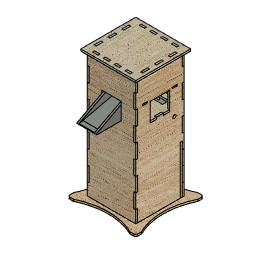
Plant fountain v41 (Autodesk Fusion 360 design; units mm, degrees)
Autodesk Fusion 360 part; units mm, degrees
(part 1 of 3)
sketch "base" plane through (0, 0, 0) normal (0, 0, 1) x (1, 0, 0) in component "base"
  line L0 (0, 0) -> (75, 0)
  line L1 (75, 0) -> (75, 75)
  line L2 (75, 75) -> (0, 75)
  line L3 (0, 75) -> (0, 0)
  line L4 (75, 37.5) -> (0, 37.5) construction
  line L5 (37.5, 75) -> (37.5, 0) construction
  line L6 (-5, 80) -> (80, 80)
  line L7 (80, 80) -> (80, -5)
  line L8 (80, -5) -> (-5, -5)
  line L9 (-5, -5) -> (-5, 80)
  line L10 (-5, 80) -> (80, -5) construction
  line L11 (80, 80) -> (-5, -5) construction
  point P0 (37.5, 37.5)
  dimension "d14" = 75
  dimension "d15" = 75
  dimension "d16" = 5
  dimension "d17" = 5
  constraint horizontal L0
  constraint vertical L1
  constraint horizontal L2
  constraint vertical L3
  constraint coincident L0.start L3.end
  constraint midpoint L1 L4.start
  constraint midpoint L3 L4.end
  constraint midpoint L2 L5.start
  constraint midpoint L0 L5.end
  constraint horizontal L6
  constraint perpendicular L6 L7
  constraint parallel L6 L8
  constraint parallel L7 L9
  constraint coincident L10 P0
  constraint coincident L11 P0
  constraint midpoint L4 P0
  measures "d14" distance of L1.end L2.end
  measures "d15" distance of L0.end L1.end
  measures "d16" distance of L2 L6
  measures "d17" distance of L1 L7
extrude "Extrude1" add sketch "base" along normal blind 3 contours L0 L1 L2 L3 | L6 L7 L8 L9 makes body 1 in component "base"
sketch "lenghttabcut" plane through (0, 0, 3) normal (0, 0, 1) x (-1, 0, 0) in component "base"
  line L0 (5, 5) -> (-80, 5)
  line L1 (-80, 5) -> (-80, -80)
  line L2 (-80, -80) -> (5, -80)
  line L3 (5, -80) -> (5, 5)
  line L4 (-8.3333, -75) -> (-16.6667, -75)
  line L5 (-16.6667, -75) -> (-16.6667, -72)
  line L6 (-16.6667, -72) -> (-8.3333, -72)
  line L7 (-8.3333, -72) -> (-8.3333, -75)
  line L8 (-75, -75) -> (0, -75)
  line L9 (0, -75) -> (0, 0)
  dimension "d20" = 8.3333
  dimension "d21" = 8.3333
  dimension "d35" = 3
  constraint horizontal L4
  constraint vertical L5
  constraint horizontal L6
  constraint vertical L7
  constraint collinear L4 L8
  measures "d20" distance of L7 L9
  measures "d21" distance of L4.start L4.end
  measures "d35" distance of L4.start L6.end
extrude "Extrude2" cut sketch "lenghttabcut" against normal blind 3 contours L4 L5 L6 L7 L8 bodies 1 in component "base"
pattern_linear "R-Pattern1" count 4 spacing 16.6667 along (1, 0, 0) of "Extrude2" in component "base"
ref_plane "WorkPlane1" through (37.5, 75, 1.5) normal (0, 1, 0) x (-1, 0, 0) in component "back"
sketch "back" plane through (30, 75, 1.5) normal (0, 1, 0) x (1, 0, 0) in component "back"
  line L0 (-30, 1.5) -> (45, 1.5)
  line L1 (45, 1.5) -> (45, -198.5)
  line L2 (45, -198.5) -> (-30, -198.5)
  line L3 (-30, -198.5) -> (-30, 1.5)
  point P0 (7.5, 1.5)
  dimension "d29" = 200
  dimension "d30" = 75
  constraint horizontal L0
  constraint vertical L1
  constraint horizontal L2
  constraint vertical L3
  constraint midpoint L0 P0
  measures "d29" distance of L0.start L2.end
  measures "d30" distance of L1.end L2.end
extrude "Extrude1'" add sketch "back" against normal blind 3 separate body makes body 2 in component "back"
sketch "heighttabcut" plane through (75, 0, 0) normal (1, 0, 0) x (0, 1, 0) in component "back"
  line L0 (75, 0) -> (75, 200)
  line L1 (75, 200) -> (72, 200)
  line L2 (72, 200) -> (72, 0)
  line L3 (72, 0) -> (75, 0)
  line L4 (72, 44.4444) -> (75, 44.4444)
  line L5 (75, 44.4444) -> (75, 22.2222)
  line L6 (75, 22.2222) -> (72, 22.2222)
  line L7 (72, 22.2222) -> (72, 44.4444)
  line L8 (80, 0) -> (-5, 0)
  dimension "d33" = 22.2222
  dimension "d34" = 22.2222
  constraint horizontal L4
  constraint vertical L5
  constraint horizontal L6
  constraint vertical L7
  constraint coincident L0 L5.end
  constraint coincident L2 L4.start
  measures "d33" distance of L6 L8
  measures "d34" distance of L4.end L5.end
combine "Combine1" operation cut target body 2 tool bodies 1 keep tools in component "back"
extrude "Extrude2'" cut sketch "heighttabcut" against normal blind 3 contours L0 L2 L4 L5 L6 L7 bodies 2 in component "back"
pattern_linear "R-Pattern1'" count 4 spacing 44.4444 along (0, 0, 1) of "Extrude2'" in component "back"
extrude "Extrude1''" add 1 faces at (24, 75, 104.7037) along direction (0, 1, 0) blind 3 from surface at -75 separate body on bodies 2 makes body 3 in component "front"
combine "Combine1'" operation cut target body 1 tool bodies 3 keep tools in component "base"
sketch "widthtabcut" plane through (0, 0, 3) normal (0, 0, 1) x (-1, 0, 0) in component "base"
  line L0 (-8.3333, 0) -> (-8.3333, -3)
  line L1 (-8.3333, -3) -> (-16.6667, -3)
  line L2 (-16.6667, -3) -> (-16.6667, 0)
  line L3 (-16.6667, 0) -> (-8.3333, 0)
  line L4 (-25, 0) -> (-25, -3)
  line L5 (-25, -3) -> (-33.3333, -3)
  line L6 (-33.3333, -3) -> (-33.3333, 0)
  line L7 (-33.3333, 0) -> (-25, 0)
  line L8 (-41.6667, 0) -> (-41.6667, -3)
  line L9 (-41.6667, -3) -> (-50, -3)
  line L10 (-50, -3) -> (-50, 0)
  line L11 (-50, 0) -> (-41.6667, 0)
  line L12 (-41.6667, -72) -> (-41.6667, -75)
  line L13 (-41.6667, -75) -> (-50, -75)
  line L14 (-50, -75) -> (-50, -72)
  line L15 (-50, -72) -> (-41.6667, -72)
  line L16 (-25, -72) -> (-25, -75)
  line L17 (-25, -75) -> (-33.3333, -75)
  line L18 (-33.3333, -75) -> (-33.3333, -72)
  line L19 (-33.3333, -72) -> (-25, -72)
  line L20 (-8.3333, -72) -> (-8.3333, -75)
  line L21 (-8.3333, -75) -> (-16.6667, -75)
  line L22 (-16.6667, -75) -> (-16.6667, -72)
  line L23 (-16.6667, -72) -> (-8.3333, -72)
  line L24 (5, 5) -> (-80, 5)
  line L25 (-80, 5) -> (-80, -80)
  line L26 (-80, -80) -> (5, -80)
  line L27 (5, -80) -> (5, 5)
  line L28 (-75, -64.2857) -> (-72, -64.2857)
  line L29 (-72, -64.2857) -> (-72, -53.5714)
  line L30 (-72, -53.5714) -> (-75, -53.5714)
  line L31 (-75, -53.5714) -> (-75, -64.2857)
  line L32 (-75, -75) -> (0, -75)
  line L33 (-75, 0) -> (-75, -75)
  line L34 (-58.3333, 0) -> (-58.3333, -3)
  line L35 (-58.3333, -3) -> (-66.6667, -3)
  line L36 (-66.6667, -3) -> (-66.6667, 0)
  line L37 (-66.6667, 0) -> (-58.3333, 0)
  line L38 (-58.3333, -72) -> (-58.3333, -75)
  line L39 (-58.3333, -75) -> (-66.6667, -75)
  line L40 (-66.6667, -75) -> (-66.6667, -72)
  line L41 (-66.6667, -72) -> (-58.3333, -72)
  dimension "d45" = 3
  dimension "d46" = 10.7143
  dimension "d47" = 10.7143
  constraint horizontal L28
  constraint vertical L29
  constraint horizontal L30
  constraint vertical L31
  constraint collinear L31 L33
  measures "d45" distance of L28.start L28.end
  measures "d46" distance of L28 L32
  measures "d47" distance of L28.start L30.end
extrude "Extrude3" cut sketch "widthtabcut" against normal blind 3 contours L28 L29 L30 L31 L33 bodies 1 in component "base"
pattern_linear "R-Pattern2" count 3 spacing 21.4286 along (0, -1, 0) of "Extrude3" in component "base"
sketch "Sketch1" plane through (75, 0, 0) normal (1, 0, 0) x (0, 1, 0) in component "right"
  line L0 (75, 177.7778) -> (75, 200)
  line L1 (75, 200) -> (72, 200)
  line L2 (72, 200) -> (72, 177.7778)
  line L3 (0, 0) -> (75, 0)
  line L4 (75, 0) -> (75, 200)
  line L5 (75, 200) -> (0, 200)
  line L6 (0, 200) -> (0, 0)
  line L7 (72, 177.7778) -> (75, 177.7778)
  constraint perpendicular L3 L4
  constraint parallel L3 L5
  constraint parallel L4 L6
  constraint horizontal L3
  constraint coincident L3.start L6.end
  constraint coincident L0.end L1.start
extrude "Extrude1'''" add sketch "Sketch1" against normal blind 3 separate body makes body 4 in component "right"
combine "Combine1''" operation cut target body 4 tool bodies 2 keep tools in component "right"
combine "Combine2" operation cut target body 4 tool bodies 3 keep tools in component "right"
combine "Combine3" operation cut target body 4 tool bodies 1 keep tools in component "right"
extrude "Extrude1''''" add 1 faces at (72, 35.7143, 30.6296) along direction (-1, 0, 0) blind 3 from surface at 69 separate body on bodies 4 makes body 5 in component "left"
combine "Combine2'" operation cut target body 2 tool bodies 5 keep tools in component "back"
combine "Combine1'''" operation cut target body 3 tool bodies 5 keep tools in component "front"
combine "Combine2''" operation cut target body 1 tool bodies 5 keep tools in component "base"
sketch "extension" plane through (0, 0, 3) normal (0, 0, 1) x (-1, 0, 0) in component "base"
  line L0 (-3, -10.7143) -> (0, -10.7143)
  line L1 (0, -10.7143) -> (0, -21.4286)
  line L2 (0, -21.4286) -> (-3, -21.4286)
  line L3 (-3, -21.4286) -> (-3, -10.7143)
  line L4 (-3, -32.1429) -> (0, -32.1429)
  line L5 (0, -32.1429) -> (0, -42.8571)
  line L6 (0, -42.8571) -> (-3, -42.8571)
  line L7 (-3, -42.8571) -> (-3, -32.1429)
  line L8 (-3, -53.5714) -> (0, -53.5714)
  line L9 (0, -53.5714) -> (0, -64.2857)
  line L10 (0, -64.2857) -> (-3, -64.2857)
  line L11 (-3, -64.2857) -> (-3, -53.5714)
  line L12 (-75, -21.4286) -> (-75, -10.7143)
  line L13 (-75, -10.7143) -> (-72, -10.7143)
  line L14 (-72, -10.7143) -> (-72, -21.4286)
  line L15 (-72, -21.4286) -> (-75, -21.4286)
  line L16 (-75, -42.8571) -> (-75, -32.1429)
  line L17 (-75, -32.1429) -> (-72, -32.1429)
  line L18 (-72, -32.1429) -> (-72, -42.8571)
  line L19 (-72, -42.8571) -> (-75, -42.8571)
  line L20 (-75, -64.2857) -> (-75, -53.5714)
  line L21 (-75, -53.5714) -> (-72, -53.5714)
  line L22 (-72, -53.5714) -> (-72, -64.2857)
  line L23 (-72, -64.2857) -> (-75, -64.2857)
  line L24 (-8.3333, 0) -> (-8.3333, -3)
  line L25 (-8.3333, -3) -> (-16.6667, -3)
  line L26 (-16.6667, -3) -> (-16.6667, 0)
  line L27 (-16.6667, 0) -> (-8.3333, 0)
  line L28 (-25, 0) -> (-25, -3)
  line L29 (-25, -3) -> (-33.3333, -3)
  line L30 (-33.3333, -3) -> (-33.3333, 0)
  line L31 (-33.3333, 0) -> (-25, 0)
  line L32 (-41.6667, 0) -> (-41.6667, -3)
  line L33 (-41.6667, -3) -> (-50, -3)
  line L34 (-50, -3) -> (-50, 0)
  line L35 (-50, 0) -> (-41.6667, 0)
  line L36 (-58.3333, 0) -> (-58.3333, -3)
  line L37 (-58.3333, -3) -> (-66.6667, -3)
  line L38 (-66.6667, -3) -> (-66.6667, 0)
  line L39 (-66.6667, 0) -> (-58.3333, 0)
  line L40 (-58.3333, -72) -> (-58.3333, -75)
  line L41 (-58.3333, -75) -> (-66.6667, -75)
  line L42 (-66.6667, -75) -> (-66.6667, -72)
  line L43 (-66.6667, -72) -> (-58.3333, -72)
  line L44 (-41.6667, -72) -> (-41.6667, -75)
  line L45 (-41.6667, -75) -> (-50, -75)
  line L46 (-50, -75) -> (-50, -72)
  line L47 (-50, -72) -> (-41.6667, -72)
  line L48 (-25, -72) -> (-25, -75)
  line L49 (-25, -75) -> (-33.3333, -75)
  line L50 (-33.3333, -75) -> (-33.3333, -72)
  line L51 (-33.3333, -72) -> (-25, -72)
  line L52 (-8.3333, -72) -> (-8.3333, -75)
  line L53 (-8.3333, -75) -> (-16.6667, -75)
  line L54 (-16.6667, -75) -> (-16.6667, -72)
  line L55 (-16.6667, -72) -> (-8.3333, -72)
  line L56 (5, 5) -> (-80, 5)
  line L57 (-80, 5) -> (-80, -80)
  line L58 (-80, -80) -> (5, -80)
  line L59 (5, -80) -> (5, 5)
  circle A0 centre (-37.5, -180) radius 100
  circle A1 centre (-180, -37.5) radius 100
  circle A2 centre (-37.5, 105) radius 100
  circle A3 centre (105, -37.5) radius 100
  line L60 (5, -80) -> (-80, -80)
  line L61 (-80, -80) -> (-80, 5)
  line L62 (-80, 5) -> (5, 5)
  line L63 (5, 5) -> (5, -80)
  line L64 (5, -37.5) -> (-80, -37.5) construction
  line L65 (-37.5, -80) -> (-37.5, 5) construction
  line L66 (-90, -90) -> (15, -90)
  line L67 (15, -90) -> (15, 15)
  line L68 (15, 15) -> (-90, 15)
  line L69 (-90, 15) -> (-90, -90)
  line L70 (-90, -90) -> (15, 15) construction
  line L71 (15, -90) -> (-90, 15) construction
  point P0 (-37.5, -37.5)
  dimension "d60" = 200
  dimension "d62" = 10
  constraint equal A0 A3
  constraint equal A0 A1
  constraint equal A0 A2
  constraint tangent A0 L60
  constraint tangent A1 L61
  constraint tangent A2 L62
  constraint tangent A3 L63
  constraint midpoint L63 L64.start
  constraint midpoint L61 L64.end
  constraint midpoint L60 L65.start
  constraint midpoint L62 L65.end
  constraint coincident A0 L65.start
  constraint coincident A3 L64.start
  constraint coincident A1 L64.end
  constraint coincident A2 L65.end
  constraint horizontal L66
  constraint perpendicular L66 L67
  constraint parallel L66 L68
  constraint parallel L67 L69
  constraint coincident L70 P0
  constraint coincident L71 P0
  constraint midpoint L64 P0
  constraint equal L66 L69
  measures "d60" diameter of A0
  measures "d62" distance of L60 L66
extrude "Extrude4" add sketch "extension" against normal blind 3 contours L56 L59 A2 A3 L62 L63 L67 L68 | L56 L57 A1 A2 L61 L62 L68 L69 | L58 L59 A0 A3 L60 L63 L66 L67 | L57 L58 A0 A1 L60 L61 L66 L69 bodies 1 in component "base"
fillet "Fillet1" radius 3 4 edges at (-15, -15, 1.5) (-15, 90, 1.5) (90, 90, 1.5) (90, -15, 1.5) on bodies 1 in component "base"
sketch "spout_cut" plane through (72, 0, 0) normal (-1, 0, 0) x (0, -1, 0) in component "right"
  line L0 (-72, 3) -> (-64.2857, 3)
  line L1 (-64.2857, 3) -> (-64.2857, 0)
  line L2 (-64.2857, 0) -> (-53.5714, 0)
  line L3 (-53.5714, 0) -> (-53.5714, 3)
  line L4 (-53.5714, 3) -> (-42.8571, 3)
  line L5 (-42.8571, 3) -> (-42.8571, 0)
  line L6 (-42.8571, 0) -> (-32.1429, 0)
  line L7 (-32.1429, 0) -> (-32.1429, 3)
  line L8 (-32.1429, 3) -> (-21.4286, 3)
  line L9 (-21.4286, 3) -> (-21.4286, 0)
  line L10 (-21.4286, 0) -> (-10.7143, 0)
  line L11 (-10.7143, 0) -> (-10.7143, 3)
  line L12 (-10.7143, 3) -> (-3, 3)
  line L13 (-3, 3) -> (-3, 22.2222)
  line L14 (-3, 22.2222) -> (0, 22.2222)
  line L15 (0, 22.2222) -> (0, 44.4444)
  line L16 (0, 44.4444) -> (-3, 44.4444)
  line L17 (-3, 44.4444) -> (-3, 66.6667)
  line L18 (-3, 66.6667) -> (0, 66.6667)
  line L19 (0, 66.6667) -> (0, 88.8889)
  line L20 (0, 88.8889) -> (-3, 88.8889)
  line L21 (-3, 88.8889) -> (-3, 111.1111)
  line L22 (-3, 111.1111) -> (0, 111.1111)
  line L23 (0, 111.1111) -> (0, 133.3333)
  line L24 (0, 133.3333) -> (-3, 133.3333)
  line L25 (-3, 133.3333) -> (-3, 155.5556)
  line L26 (-3, 155.5556) -> (0, 155.5556)
  line L27 (0, 155.5556) -> (0, 177.7778)
  line L28 (0, 177.7778) -> (-3, 177.7778)
  line L29 (-3, 177.7778) -> (-3, 200)
  line L30 (-3, 200) -> (-72, 200)
  line L31 (-72, 200) -> (-72, 177.7778)
  line L32 (-72, 177.7778) -> (-75, 177.7778)
  line L33 (-75, 177.7778) -> (-75, 155.5556)
  line L34 (-75, 155.5556) -> (-72, 155.5556)
  line L35 (-72, 155.5556) -> (-72, 133.3333)
  line L36 (-72, 133.3333) -> (-75, 133.3333)
  line L37 (-75, 133.3333) -> (-75, 111.1111)
  line L38 (-75, 111.1111) -> (-72, 111.1111)
  line L39 (-72, 111.1111) -> (-72, 88.8889)
  line L40 (-72, 88.8889) -> (-75, 88.8889)
  line L41 (-75, 88.8889) -> (-75, 66.6667)
  line L42 (-75, 66.6667) -> (-72, 66.6667)
  line L43 (-72, 66.6667) -> (-72, 44.4444)
  line L44 (-72, 44.4444) -> (-75, 44.4444)
  line L45 (-75, 44.4444) -> (-75, 22.2222)
  line L46 (-75, 22.2222) -> (-72, 22.2222)
  line L47 (-72, 22.2222) -> (-72, 3)
  line L48 (-52.5, 200) -> (-22.5, 200)
  line L49 (-22.5, 200) -> (-22.5, 130)
  line L50 (-22.5, 130) -> (-52.5, 130)
  line L51 (-52.5, 130) -> (-52.5, 200)
  dimension "d69" = 70
  dimension "d70" = 30
  constraint horizontal L48
  constraint vertical L49
  constraint horizontal L50
  constraint vertical L51
  constraint coincident L30 L48.start
  constraint midpoint L30 L48
  measures "d69" distance of L48.end L49.end
  measures "d70" distance of L49.end L50.end
extrude "Extrude2''" cut sketch "spout_cut" against normal blind 10 contours L30 L48 L49 L50 L51 bodies 4 in component "right"
sketch "spout_cut (2)" plane through (0, 0, 0) normal (-1, 0, 0) x (0, -1, 0) in component "left"
  line L0 (-72, 22.2222) -> (-72, 3)
  line L1 (-72, 3) -> (-64.2857, 3)
  line L2 (-64.2857, 3) -> (-64.2857, 0)
  line L3 (-64.2857, 0) -> (-53.5714, 0)
  line L4 (-53.5714, 0) -> (-53.5714, 3)
  line L5 (-53.5714, 3) -> (-42.8571, 3)
  line L6 (-42.8571, 3) -> (-42.8571, 0)
  line L7 (-42.8571, 0) -> (-32.1429, 0)
  line L8 (-32.1429, 0) -> (-32.1429, 3)
  line L9 (-32.1429, 3) -> (-21.4286, 3)
  line L10 (-21.4286, 3) -> (-21.4286, 0)
  line L11 (-21.4286, 0) -> (-10.7143, 0)
  line L12 (-10.7143, 0) -> (-10.7143, 3)
  line L13 (-10.7143, 3) -> (-3, 3)
  line L14 (-3, 3) -> (-3, 22.2222)
  line L15 (-3, 22.2222) -> (0, 22.2222)
  line L16 (0, 22.2222) -> (0, 44.4444)
  line L17 (0, 44.4444) -> (-3, 44.4444)
  line L18 (-3, 44.4444) -> (-3, 66.6667)
  line L19 (-3, 66.6667) -> (0, 66.6667)
  line L20 (0, 66.6667) -> (0, 88.8889)
  line L21 (0, 88.8889) -> (-3, 88.8889)
  line L22 (-3, 88.8889) -> (-3, 111.1111)
  line L23 (-3, 111.1111) -> (0, 111.1111)
  line L24 (0, 111.1111) -> (0, 133.3333)
  line L25 (0, 133.3333) -> (-3, 133.3333)
  line L26 (-3, 133.3333) -> (-3, 155.5556)
  line L27 (-3, 155.5556) -> (0, 155.5556)
  line L28 (0, 155.5556) -> (0, 177.7778)
  line L29 (0, 177.7778) -> (-3, 177.7778)
  line L30 (-3, 177.7778) -> (-3, 200)
  line L31 (-3, 200) -> (-72, 200)
  line L32 (-72, 200) -> (-72, 177.7778)
  line L33 (-72, 177.7778) -> (-75, 177.7778)
  line L34 (-75, 177.7778) -> (-75, 155.5556)
  line L35 (-75, 155.5556) -> (-72, 155.5556)
  line L36 (-72, 155.5556) -> (-72, 133.3333)
  line L37 (-72, 133.3333) -> (-75, 133.3333)
  line L38 (-75, 133.3333) -> (-75, 111.1111)
  line L39 (-75, 111.1111) -> (-72, 111.1111)
  line L40 (-72, 111.1111) -> (-72, 88.8889)
  line L41 (-72, 88.8889) -> (-75, 88.8889)
  line L42 (-75, 88.8889) -> (-75, 66.6667)
  line L43 (-75, 66.6667) -> (-72, 66.6667)
  line L44 (-72, 66.6667) -> (-72, 44.4444)
  line L45 (-72, 44.4444) -> (-75, 44.4444)
  line L46 (-75, 44.4444) -> (-75, 22.2222)
  line L47 (-75, 22.2222) -> (-72, 22.2222)
  line L48 (-52.5, 200) -> (-22.5, 200)
  line L49 (-22.5, 200) -> (-22.5, 130)
  line L50 (-22.5, 130) -> (-52.5, 130)
  line L51 (-52.5, 130) -> (-52.5, 200)
  dimension "d73" = 30
  dimension "d74" = 70
  constraint horizontal L48
  constraint vertical L49
  constraint horizontal L50
  constraint vertical L51
  constraint midpoint L31 L48
  measures "d73" distance of L49.end L50.end
  measures "d74" distance of L48.end L49.end
extrude "Extrude2'''" cut sketch "spout_cut (2)" against normal blind 5 contours L31 L48 L49 L50 L51 bodies 5 in component "left"
sketch "spout_cut (3)" plane through (0, 0, 0) normal (0, -1, 0) x (1, 0, 0) in component "front"
  line L0 (3, 22.2222) -> (0, 22.2222)
  line L1 (0, 22.2222) -> (0, 3)
  line L2 (0, 3) -> (8.3333, 3)
  line L3 (8.3333, 3) -> (8.3333, 0)
  line L4 (8.3333, 0) -> (16.6667, 0)
  line L5 (16.6667, 0) -> (16.6667, 3)
  line L6 (16.6667, 3) -> (25, 3)
  line L7 (25, 3) -> (25, 0)
  line L8 (25, 0) -> (33.3333, 0)
  line L9 (33.3333, 0) -> (33.3333, 3)
  line L10 (33.3333, 3) -> (41.6667, 3)
  line L11 (41.6667, 3) -> (41.6667, 0)
  line L12 (41.6667, 0) -> (50, 0)
  line L13 (50, 0) -> (50, 3)
  line L14 (50, 3) -> (58.3333, 3)
  line L15 (58.3333, 3) -> (58.3333, 0)
  line L16 (58.3333, 0) -> (66.6667, 0)
  line L17 (66.6667, 0) -> (66.6667, 3)
  line L18 (66.6667, 3) -> (75, 3)
  line L19 (75, 3) -> (75, 22.2222)
  line L20 (75, 22.2222) -> (72, 22.2222)
  line L21 (72, 22.2222) -> (72, 44.4444)
  line L22 (72, 44.4444) -> (75, 44.4444)
  line L23 (75, 44.4444) -> (75, 66.6667)
  line L24 (75, 66.6667) -> (72, 66.6667)
  line L25 (72, 66.6667) -> (72, 88.8889)
  line L26 (72, 88.8889) -> (75, 88.8889)
  line L27 (75, 88.8889) -> (75, 111.1111)
  line L28 (75, 111.1111) -> (72, 111.1111)
  line L29 (72, 111.1111) -> (72, 133.3333)
  line L30 (72, 133.3333) -> (75, 133.3333)
  line L31 (75, 133.3333) -> (75, 155.5556)
  line L32 (75, 155.5556) -> (72, 155.5556)
  line L33 (72, 155.5556) -> (72, 177.7778)
  line L34 (72, 177.7778) -> (75, 177.7778)
  line L35 (75, 177.7778) -> (75, 200)
  line L36 (75, 200) -> (0, 200)
  line L37 (0, 200) -> (0, 177.7778)
  line L38 (0, 177.7778) -> (3, 177.7778)
  line L39 (3, 177.7778) -> (3, 155.5556)
  line L40 (3, 155.5556) -> (0, 155.5556)
  line L41 (0, 155.5556) -> (0, 133.3333)
  line L42 (0, 133.3333) -> (3, 133.3333)
  line L43 (3, 133.3333) -> (3, 111.1111)
  line L44 (3, 111.1111) -> (0, 111.1111)
  line L45 (0, 111.1111) -> (0, 88.8889)
  line L46 (0, 88.8889) -> (3, 88.8889)
  line L47 (3, 88.8889) -> (3, 66.6667)
  line L48 (3, 66.6667) -> (0, 66.6667)
  line L49 (0, 66.6667) -> (0, 44.4444)
  line L50 (0, 44.4444) -> (3, 44.4444)
  line L51 (3, 44.4444) -> (3, 22.2222)
  line L52 (22.5, 200) -> (52.5, 200)
  line L53 (52.5, 200) -> (52.5, 130)
  line L54 (52.5, 130) -> (22.5, 130)
  line L55 (22.5, 130) -> (22.5, 200)
  dimension "d77" = 30
  dimension "d78" = 70
  constraint horizontal L52
  constraint vertical L53
  constraint horizontal L54
  constraint vertical L55
  constraint midpoint L36 L52
  measures "d77" distance of L53.end L54.end
  measures "d78" distance of L52.end L53.end
extrude "Extrude2''''" cut sketch "spout_cut (3)" against normal blind 5 contours L36 L52 L53 L54 L55 bodies 3 in component "front"
sketch "Sketch1 (2)" plane through (0, 0, 130) normal (0, 0, 1) x (-1, 0, 0) in component "mid panel"
  line L0 (-75, -22.5) -> (-75, -52.5)
  line L1 (-75, -52.5) -> (-72, -52.5)
  line L2 (-72, -52.5) -> (-72, -22.5)
  line L3 (-72, -22.5) -> (-75, -22.5)
  line L4 (0, -75) -> (-75, -75)
  line L5 (-75, -75) -> (-75, 0)
  line L6 (-75, 0) -> (0, 0)
  line L7 (0, 0) -> (0, -75)
  line L8 (-52.5, 0) -> (-75, 0)
  line L9 (-8.3333, -75) -> (-16.6667, -75)
  line L10 (-16.6667, -75) -> (-16.6667, -72)
  line L11 (-16.6667, -72) -> (-8.3333, -72)
  line L12 (-8.3333, -72) -> (-8.3333, -75)
  line L13 (-25, -72) -> (-33.3333, -72)
  line L14 (-33.3333, -72) -> (-33.3333, -75)
  line L15 (-33.3333, -75) -> (-25, -75)
  line L16 (-25, -75) -> (-25, -72)
  line L17 (-41.6667, -75) -> (-50, -75)
  line L18 (-50, -75) -> (-50, -72)
  line L19 (-50, -72) -> (-41.6667, -72)
  line L20 (-41.6667, -72) -> (-41.6667, -75)
  line L21 (-58.3333, -75) -> (-66.6667, -75)
  line L22 (-66.6667, -75) -> (-66.6667, -72)
  line L23 (-66.6667, -72) -> (-58.3333, -72)
  line L24 (-58.3333, -72) -> (-58.3333, -75)
  line L25 (-75, -64.2857) -> (-72, -64.2857)
  line L26 (-72, -64.2857) -> (-72, -53.5714)
  line L27 (-72, -53.5714) -> (-75, -53.5714)
  line L28 (-75, -53.5714) -> (-75, -64.2857)
  line L29 (-75, -42.8571) -> (-72, -42.8571)
  line L30 (-72, -42.8571) -> (-72, -32.1429)
  line L31 (-72, -32.1429) -> (-75, -32.1429)
  line L32 (-75, -32.1429) -> (-75, -42.8571)
  line L33 (-75, -10.7143) -> (-75, -21.233)
  line L34 (-75, -21.4286) -> (-72, -21.4286)
  line L35 (-72, -21.4286) -> (-72, -10.7143)
  line L36 (-72, -10.7143) -> (-75, -10.7143)
  line L37 (-75, -10.7143) -> (-75, -21.4286)
  line L38 (-75, -3) -> (-72, -3)
  line L39 (0, -37.5) -> (-75, -37.5)
  line L40 (-37.5, 0) -> (-37.5, -75)
  line L41 (-66.6667, 0) -> (-66.6667, -3)
  line L42 (-41.6667, 0) -> (-50, 0)
  line L43 (-41.6667, -3) -> (-41.6667, 0)
  line L44 (-8.3333, 0) -> (-16.6667, 0)
  line L45 (-58.3333, 0) -> (-66.6667, 0)
  line L46 (-66.6667, -3) -> (-58.3333, -3)
  line L47 (-33.3333, -3) -> (-33.3333, 0)
  line L48 (-50, 0) -> (-50, -3)
  line L49 (-25, 0) -> (-25, -3)
  line L50 (-58.3333, -3) -> (-58.3333, 0)
  line L51 (-16.6667, -3) -> (-8.3333, -3)
  line L52 (-8.3333, -3) -> (-8.3333, 0)
  line L53 (-25, -3) -> (-33.3333, -3)
  line L54 (-16.6667, 0) -> (-16.6667, -3)
  line L55 (-50, -3) -> (-41.6667, -3)
  line L56 (-33.3333, 0) -> (-25, 0)
  line L57 (-3, -32.1429) -> (0, -32.1429)
  line L58 (0, -10.7143) -> (0, -21.233)
  line L59 (0, -32.1429) -> (0, -42.8571)
  line L60 (0, -21.4286) -> (-3, -21.4286)
  line L61 (0, -42.8571) -> (-3, -42.8571)
  line L62 (0, -22.5) -> (0, -52.5)
  line L63 (-3, -42.8571) -> (-3, -32.1429)
  line L64 (0, -52.5) -> (-3, -52.5)
  line L65 (-3, -22.5) -> (0, -22.5)
  line L66 (0, -64.2857) -> (-3, -64.2857)
  line L67 (-3, -52.5) -> (-3, -22.5)
  line L68 (-3, -10.7143) -> (0, -10.7143)
  line L69 (-3, -53.5714) -> (0, -53.5714)
  line L70 (0, -53.5714) -> (0, -64.2857)
  line L71 (-3, -64.2857) -> (-3, -53.5714)
  line L72 (0, -3) -> (-3, -3)
  line L73 (0, -10.7143) -> (0, -21.4286)
  line L74 (-3, -21.4286) -> (-3, -10.7143)
  line L75 (-3, -3) -> (-72, -3)
  line L76 (-72, -3) -> (-72, -72)
  line L77 (-72, -72) -> (-3, -72)
  line L78 (-3, -72) -> (-3, -3)
  line L79 (-3, -3) -> (-72, -72) construction
  line L80 (-72, -3) -> (-3, -72) construction
  point P0 (0, -75)
  point P1 (-37.5, 0)
  point P2 (0, -37.5)
  point P3 (-37.5, -37.5)
  dimension "d81" = 10.7143
  dimension "d82" = 8.3333
  dimension "d83" = 3
  dimension "d84" = 8.3333
  dimension "d85" = 8.3333
  dimension "d86" = 8.3333
  dimension "d87" = 8.3333
  dimension "d88" = 3
  dimension "d89" = 10.7143
  dimension "d90" = 10.7143
  dimension "d94" = 10.7143
  constraint horizontal L4
  constraint vertical L5
  constraint horizontal L6
  constraint vertical L7
  constraint coincident P0 L4.start
  constraint coincident L5.end L8
  constraint coincident L5.end L6.start
  constraint horizontal L9
  constraint vertical L10
  constraint horizontal L11
  constraint vertical L12
  constraint coincident L4 L9.start
  constraint horizontal L13
  constraint vertical L14
  constraint horizontal L15
  constraint vertical L16
  constraint coincident L4 L14.end
  constraint horizontal L17
  constraint vertical L18
  constraint horizontal L19
  constraint vertical L20
  constraint coincident L4 L17.start
  constraint horizontal L21
  constraint vertical L22
  constraint horizontal L23
  constraint vertical L24
  constraint coincident L4 L21.start
  constraint horizontal L25
  constraint vertical L26
  constraint horizontal L27
  constraint vertical L28
  constraint coincident L5 L25.start
  constraint horizontal L29
  constraint vertical L30
  constraint horizontal L31
  constraint vertical L32
  constraint coincident L2 L30.end
  constraint coincident L5 L29.start
  constraint vertical L33
  constraint coincident L5 L33.end
  constraint equal L11 L23
  constraint equal L13 L23
  constraint equal L19 L23
  constraint equal L18 L22
  constraint equal L14 L22
  constraint equal L10 L22
  constraint equal L26 L30
  constraint horizontal L34
  constraint vertical L35
  constraint horizontal L36
  constraint vertical L37
  constraint coincident L5 L34.start
  constraint equal L26 L35
  constraint equal L25 L34
  constraint midpoint L7 P2
  constraint midpoint L32 L39.end
  constraint midpoint L6 P1
  constraint midpoint L4 L40.end
  constraint symmetric L9.start L39 L44.start
  constraint symmetric L9.end L39 L44.end
  constraint symmetric L10.end L39 L51.start
  constraint symmetric L11.end L39 L51.end
  constraint symmetric L13.start L39 L49.end
  constraint symmetric L13.end L39 L47.start
  constraint symmetric L14.end L39 L47.end
  constraint symmetric L15.end L39 L49.start
  constraint symmetric L17.start L39 L42.start
  constraint symmetric L17.end L39 L42.end
  constraint symmetric L18.end L39 L48.end
  constraint symmetric L19.end L39 L43.start
  constraint symmetric L21.start L39 L45.start
  constraint symmetric L21.end L39 L41.start
  constraint symmetric L22.end L39 L41.end
  constraint symmetric L23.end L39 L46.end
  constraint symmetric L39 L40.end P1
  constraint symmetric L0.start L40 L62.start
  constraint symmetric L0.end L40 L62.end
  constraint symmetric L1.end L40 L64.end
  constraint symmetric L2.end L40 L65.start
  constraint symmetric L25.start L40 L66.start
  constraint symmetric L25.end L40 L66.end
  constraint symmetric L26.end L40 L69.start
  constraint symmetric L27.end L40 L69.end
  constraint symmetric L29.start L40 L59.end
  constraint symmetric L29.end L40 L61.end
  constraint symmetric L30.end L40 L57.start
  constraint symmetric L31.end L40 L57.end
  constraint symmetric L33.end L40 L58.end
  constraint symmetric L33.start L40 L58.start
  constraint symmetric L34.start L40 L60.start
  constraint symmetric L34.end L40 L60.end
  constraint symmetric L35.end L40 L68.start
  constraint symmetric L38.start L40 L72.start
  constraint symmetric L38.end L40 L72.end
  constraint symmetric L39.end L40 P2
  constraint horizontal L75
  constraint perpendicular L75 L76
  constraint parallel L75 L77
  constraint parallel L76 L78
  constraint coincident L79 P3
  constraint coincident L80 P3
  constraint midpoint L39 P3
  measures "d81" distance of L25.end L26.end
  measures "d82" distance of L22.end L23.end
  measures "d83" distance of L21.end L22.end
  measures "d84" distance of L18 L24
  measures "d85" distance of L14 L20
  measures "d86" distance of L10 L16
  measures "d87" distance of L7 L12
  measures "d88" distance of L25.start L25.end
  measures "d89" distance of L27 L29
  measures "d90" distance of L31 L34
  measures "d94" distance of L6 L36
extrude "Extrude3'" cut sketch "Sketch1 (2)" against normal blind 3 contours L0 L2 L3 L5 L31 L76 | L0 L1 L2 L5 L29 L76 | L7 L61 L62 L64 L67 L78 | L7 L57 L62 L65 L67 L78 | L6 L47 L49 L53 L56 L75 | L6 L42 L43 L48 L55 L75 bodies 3 in component "front"
extrude "Extrude3''" cut sketch "Sketch1 (2)" against normal blind 3 contours L0 L2 L3 L5 L31 L76 | L0 L1 L2 L5 L29 L76 | L7 L61 L62 L64 L67 L78 | L7 L57 L62 L65 L67 L78 | L6 L47 L49 L53 L56 L75 | L6 L42 L43 L48 L55 L75 bodies 4 in component "right"
extrude "Extrude3'''" cut sketch "Sketch1 (2)" against normal blind 3 contours L0 L2 L3 L5 L31 L76 | L0 L1 L2 L5 L29 L76 | L7 L61 L62 L64 L67 L78 | L7 L57 L62 L65 L67 L78 | L6 L47 L49 L53 L56 L75 | L6 L42 L43 L48 L55 L75 bodies 5 in component "left"
extrude "Extrude4'" add sketch "Sketch1 (2)" against normal blind 3 separate body contours L0 L2 L3 L5 L31 L76 | L2 L30 L35 L39 L40 L46 L55 L75 L76 | L0 L1 L2 L5 L29 L76 | L2 L19 L23 L26 L30 L39 L40 L76 L77 | L39 L40 L51 L53 L63 L67 L74 L75 L78 | L11 L13 L39 L40 L63 L67 L71 L77 L78 | L7 L61 L62 L64 L67 L78 | L7 L57 L62 L65 L67 L78 | L6 L47 L49 L53 L56 L75 | L6 L42 L43 L48 L55 L75 makes body 6 in component "mid panel"
combine "Combine4" operation cut target body 3 tool bodies 6 keep tools in component "front"
combine "Combine2'''" operation cut target body 5 tool bodies 6 keep tools in component "left"
combine "Combine5" operation cut target body 4 tool bodies 6 keep tools in component "right"
sketch "Sketch4" plane through (0, 75, 0) normal (0, 1, 0) x (-1, 0, 0) in component "back"
  line L0 (0, 22.2222) -> (-3, 22.2222)
  line L1 (-3, 22.2222) -> (-3, 44.4444)
  line L2 (-3, 44.4444) -> (0, 44.4444)
  line L3 (0, 44.4444) -> (0, 66.6667)
  line L4 (0, 66.6667) -> (-3, 66.6667)
  line L5 (-3, 66.6667) -> (-3, 88.8889)
  line L6 (-3, 88.8889) -> (0, 88.8889)
  line L7 (0, 88.8889) -> (0, 111.1111)
  line L8 (0, 111.1111) -> (-3, 111.1111)
  line L9 (-3, 111.1111) -> (-3, 133.3333)
  line L10 (-3, 133.3333) -> (0, 133.3333)
  line L11 (0, 133.3333) -> (0, 155.5556)
  line L12 (0, 155.5556) -> (-3, 155.5556)
  line L13 (-3, 155.5556) -> (-3, 177.7778)
  line L14 (-3, 177.7778) -> (0, 177.7778)
  line L15 (0, 177.7778) -> (0, 200)
  line L16 (0, 200) -> (-75, 200)
  line L17 (-75, 200) -> (-75, 177.7778)
  line L18 (-75, 177.7778) -> (-72, 177.7778)
  line L19 (-72, 177.7778) -> (-72, 155.5556)
  line L20 (-72, 155.5556) -> (-75, 155.5556)
  line L21 (-75, 155.5556) -> (-75, 133.3333)
  line L22 (-75, 133.3333) -> (-72, 133.3333)
  line L23 (-72, 133.3333) -> (-72, 111.1111)
  line L24 (-72, 111.1111) -> (-75, 111.1111)
  line L25 (-75, 111.1111) -> (-75, 88.8889)
  line L26 (-75, 88.8889) -> (-72, 88.8889)
  line L27 (-72, 88.8889) -> (-72, 66.6667)
  line L28 (-72, 66.6667) -> (-75, 66.6667)
  line L29 (-75, 66.6667) -> (-75, 44.4444)
  line L30 (-75, 44.4444) -> (-72, 44.4444)
  line L31 (-72, 44.4444) -> (-72, 22.2222)
  line L32 (-72, 22.2222) -> (-75, 22.2222)
  line L33 (-75, 22.2222) -> (-75, 3)
  line L34 (-75, 3) -> (-66.6667, 3)
  line L35 (-66.6667, 3) -> (-66.6667, 0)
  line L36 (-66.6667, 0) -> (-58.3333, 0)
  line L37 (-58.3333, 0) -> (-58.3333, 3)
  line L38 (-58.3333, 3) -> (-50, 3)
  line L39 (-50, 3) -> (-50, 0)
  line L40 (-50, 0) -> (-41.6667, 0)
  line L41 (-41.6667, 0) -> (-41.6667, 3)
  line L42 (-41.6667, 3) -> (-33.3333, 3)
  line L43 (-33.3333, 3) -> (-33.3333, 0)
  line L44 (-33.3333, 0) -> (-25, 0)
  line L45 (-25, 0) -> (-25, 3)
  line L46 (-25, 3) -> (-16.6667, 3)
  line L47 (-16.6667, 3) -> (-16.6667, 0)
  line L48 (-16.6667, 0) -> (-8.3333, 0)
  line L49 (-8.3333, 0) -> (-8.3333, 3)
  line L50 (-8.3333, 3) -> (0, 3)
  line L51 (0, 3) -> (0, 22.2222)
  line L52 (-62, 78) -> (-13, 78)
  line L53 (-13, 78) -> (-13, 8)
  line L54 (-13, 8) -> (-62, 8)
  line L55 (-62, 8) -> (-62, 78)
  line L56 (-37.5, 78) -> (-37.5, 8) construction
  line L57 (-37.5, 3) -> (-37.5, 30) construction
  line L58 (-75, 44.4444) -> (-72, 44.4444)
  line L59 (-72, 44.4444) -> (-72, 22.2222)
  line L60 (-72, 22.2222) -> (-75, 22.2222)
  line L61 (-75, 22.2222) -> (-75, 44.4444)
  dimension "d114" = 8
  dimension "d116" = 10
  dimension "d117" = 70
  constraint horizontal L52
  constraint vertical L53
  constraint horizontal L54
  constraint vertical L55
  constraint midpoint L52 L56.start
  constraint midpoint L54 L56.end
  constraint midpoint L42 L57.start
  constraint perpendicular L42 L57
  constraint coincident L56 L57.end
  constraint horizontal L58
  constraint vertical L59
  constraint horizontal L60
  constraint vertical L61
  constraint coincident L31.end L32.start
  constraint coincident L29.end L30.start
  measures "d114" distance of L44 L54
  measures "d116" distance of L1 L53
  measures "d117" distance of L52.start L54.end
extrude "Extrude3''''" cut sketch "Sketch4" against normal blind 10 contours L52 L53 L54 L55 bodies 2 in component "back"
pattern_linear "R-Pattern3" count 2 spacing 6 along (0, -1, 0) of "Extrude2" in component "base"
pattern_linear "R-Pattern4" count 4 spacing 16.6667 along (1, 0, 0) of "R-Pattern3" in component "base"
sketch "Sketch1 (3)" plane through (0, 66, 0) normal (0, 1, 0) x (-1, 0, 0) in component "slider guide"
  line L0 (-58.3333, 3) -> (-66.6667, 3)
  line L1 (-66.6667, 3) -> (-66.6667, 0)
  line L2 (-66.6667, 0) -> (-58.3333, 0)
  line L3 (-58.3333, 0) -> (-58.3333, 3)
  line L4 (-72, 0) -> (-3, 0)
  line L5 (-3, 0) -> (-3, 8)
  line L6 (-3, 8) -> (-72, 8)
  line L7 (-72, 8) -> (-72, 0)
  line L8 (-3, 0) -> (-3, 3)
  line L9 (-72, 3) -> (-72, 0)
  dimension "d128" = 8
  constraint horizontal L4
  constraint vertical L5
  constraint horizontal L6
  constraint vertical L7
  constraint coincident L4.end L8
  constraint coincident L4.start L9
  measures "d128" distance of L4.end L5.end
extrude "Extrude1'''''" add sketch "Sketch1 (3)" along normal blind 3 separate body makes body 7 in component "slider guide"
combine "Combine1''''" operation cut target body 7 tool bodies 1 keep tools in component "slider guide"
sketch "Sketch4 (2)" plane through (75, 0, 0) normal (1, 0, 0) x (0, 1, 0) in component "right"
  line L0 (52.5, 200) -> (52.5, 127)
  line L1 (52.5, 127) -> (42.8571, 127)
  line L2 (42.8571, 127) -> (42.8571, 130)
  line L3 (42.8571, 130) -> (32.1429, 130)
  line L4 (32.1429, 130) -> (32.1429, 127)
  line L5 (32.1429, 127) -> (22.5, 127)
  line L6 (22.5, 127) -> (22.5, 200)
  line L7 (22.5, 200) -> (3, 200)
  line L8 (3, 200) -> (3, 177.7778)
  line L9 (3, 177.7778) -> (0, 177.7778)
  line L10 (0, 177.7778) -> (0, 155.5556)
  line L11 (0, 155.5556) -> (3, 155.5556)
  line L12 (3, 155.5556) -> (3, 133.3333)
  line L13 (3, 133.3333) -> (0, 133.3333)
  line L14 (0, 133.3333) -> (0, 111.1111)
  line L15 (0, 111.1111) -> (3, 111.1111)
  line L16 (3, 111.1111) -> (3, 88.8889)
  line L17 (3, 88.8889) -> (0, 88.8889)
  line L18 (0, 88.8889) -> (0, 66.6667)
  line L19 (0, 66.6667) -> (3, 66.6667)
  line L20 (3, 66.6667) -> (3, 44.4444)
  line L21 (3, 44.4444) -> (0, 44.4444)
  line L22 (0, 44.4444) -> (0, 22.2222)
  line L23 (0, 22.2222) -> (3, 22.2222)
  line L24 (3, 22.2222) -> (3, 3)
  line L25 (3, 3) -> (10.7143, 3)
  line L26 (10.7143, 3) -> (10.7143, 0)
  line L27 (10.7143, 0) -> (21.4286, 0)
  line L28 (21.4286, 0) -> (21.4286, 3)
  line L29 (21.4286, 3) -> (32.1429, 3)
  line L30 (32.1429, 3) -> (32.1429, 0)
  line L31 (32.1429, 0) -> (42.8571, 0)
  line L32 (42.8571, 0) -> (42.8571, 3)
  line L33 (42.8571, 3) -> (53.5714, 3)
  line L34 (53.5714, 3) -> (53.5714, 0)
  line L35 (53.5714, 0) -> (64.2857, 0)
  line L36 (64.2857, 0) -> (64.2857, 3)
  line L37 (64.2857, 3) -> (72, 3)
  line L38 (72, 3) -> (72, 22.2222)
  line L39 (72, 22.2222) -> (75, 22.2222)
  line L40 (75, 22.2222) -> (75, 44.4444)
  line L41 (75, 44.4444) -> (72, 44.4444)
  line L42 (72, 44.4444) -> (72, 66.6667)
  line L43 (72, 66.6667) -> (75, 66.6667)
  line L44 (75, 66.6667) -> (75, 88.8889)
  line L45 (75, 88.8889) -> (72, 88.8889)
  line L46 (72, 88.8889) -> (72, 111.1111)
  line L47 (72, 111.1111) -> (75, 111.1111)
  line L48 (75, 111.1111) -> (75, 133.3333)
  line L49 (75, 133.3333) -> (72, 133.3333)
  line L50 (72, 133.3333) -> (72, 155.5556)
  line L51 (72, 155.5556) -> (75, 155.5556)
  line L52 (75, 155.5556) -> (75, 177.7778)
  line L53 (75, 177.7778) -> (72, 177.7778)
  line L54 (72, 177.7778) -> (72, 200)
  line L55 (72, 200) -> (52.5, 200)
  line L56 (75, 44.4444) -> (72, 44.4444)
  line L57 (72, 44.4444) -> (72, 22.2222)
  line L58 (72, 22.2222) -> (75, 22.2222)
  line L59 (75, 22.2222) -> (75, 44.4444)
  constraint horizontal L56
  constraint vertical L57
  constraint horizontal L58
  constraint vertical L59
  constraint coincident L38.end L39.start
  constraint coincident L40.end L41.start
extrude "Extrude5" cut sketch "Sketch4 (2)" against normal blind 3 contours L39 L40 L41 L56 L57 L58 L59 bodies 2 in component "back"
extrude "Extrude5'" cut sketch "Sketch4 (2)" against normal blind 3 contours L39 L40 L41 L56 L57 L58 L59 bodies 4 in component "right"
extrude "Extrude6" add sketch "Sketch4" against normal blind 3 contours L30 L31 L32 L58 L59 L60 L61 bodies 2 in component "back"
sketch "Sketch1 (4)" plane through (0, 69, 0) normal (0, 1, 0) x (-1, 0, 0) in component "slide door"
  line L0 (-72, 3) -> (-66.6667, 3)
  line L1 (-66.6667, 3) -> (-66.6667, 0)
  line L2 (-66.6667, 0) -> (-58.3333, 0)
  line L3 (-58.3333, 0) -> (-58.3333, 3)
  line L4 (-58.3333, 3) -> (-50, 3)
  line L5 (-50, 3) -> (-50, 0)
  line L6 (-50, 0) -> (-41.6667, 0)
  line L7 (-41.6667, 0) -> (-41.6667, 3)
  line L8 (-41.6667, 3) -> (-33.3333, 3)
  line L9 (-33.3333, 3) -> (-33.3333, 0)
  line L10 (-33.3333, 0) -> (-25, 0)
  line L11 (-25, 0) -> (-25, 3)
  line L12 (-25, 3) -> (-16.6667, 3)
  line L13 (-16.6667, 3) -> (-16.6667, 0)
  line L14 (-16.6667, 0) -> (-8.3333, 0)
  line L15 (-8.3333, 0) -> (-8.3333, 3)
  line L16 (-8.3333, 3) -> (-3, 3)
  line L17 (-3, 3) -> (-3, 8)
  line L18 (-3, 8) -> (-72, 8)
  line L19 (-72, 8) -> (-72, 3)
  line L20 (-75, 3) -> (-3, 3)
  line L21 (-3, 29) -> (-18, 29) construction
  circle A0 centre (-18, 29) radius 5
  line L22 (-3, 3) -> (-3, 78)
  line L23 (-3, 78) -> (-75, 78)
  line L24 (-75, 78) -> (-75, 3)
  line L25 (-38, 34) -> (-18, 34)
  line L26 (-18, 34) -> (-18, 24)
  line L27 (-18, 24) -> (-38, 24)
  line L28 (-38, 24) -> (-38, 34)
  point P0 (-13, 78)
  point P1 (-75, 3)
  point P2 (-75, 3)
  dimension "d146" = 15
  dimension "d179" = 10
  dimension "d180" = 20
  dimension "d182" = 26
  constraint horizontal L20
  constraint coincident L16.end L17.start
  constraint coincident L21.end A0.centre
  constraint vertical L22
  constraint perpendicular L22 L23
  constraint coincident L23 P0
  constraint perpendicular L23 L24
  constraint horizontal L25
  constraint vertical L26
  constraint horizontal L27
  constraint vertical L28
  constraint coincident L21.end L26
  constraint midpoint L21.end L26
  constraint coincident L21.start L22
  constraint perpendicular L21 L22
  constraint tangent A0 L25
  measures "d146" distance of L21.start L21.end
  measures "d179" distance of L25.end L26.end
  measures "d180" distance of L25.start L25.end
  measures "d182" distance of L20 L21
extrude "Extrude1''''''" add sketch "Sketch1 (4)" along normal blind 3 separate body contours L0 L4 L8 L12 L16 L17 L18 L19 L20 L22 | L18 L19 L20 L22 L23 L24 makes body 8 in component "slide door"
sketch "Sketch3" plane through (0, 0, 130) normal (0, 0, 1) x (-1, 0, 0) in component "mid panel"
  line L0 (-75, -52.5) -> (-72, -52.5)
  line L1 (-72, -52.5) -> (-72, -72)
  line L2 (-72, -72) -> (-3, -72)
  line L3 (-3, -72) -> (-3, -52.5)
  line L4 (-3, -52.5) -> (0, -52.5)
  line L5 (0, -52.5) -> (0, -42.8571)
  line L6 (0, -42.8571) -> (-3, -42.8571)
  line L7 (-3, -42.8571) -> (-3, -32.1429)
  line L8 (-3, -32.1429) -> (0, -32.1429)
  line L9 (0, -32.1429) -> (0, -22.5)
  line L10 (0, -22.5) -> (-3, -22.5)
  line L11 (-3, -22.5) -> (-3, -3)
  line L12 (-3, -3) -> (-25, -3)
  line L13 (-25, -3) -> (-25, 0)
  line L14 (-25, 0) -> (-33.3333, 0)
  line L15 (-33.3333, 0) -> (-33.3333, -3)
  line L16 (-33.3333, -3) -> (-41.6667, -3)
  line L17 (-41.6667, -3) -> (-41.6667, 0)
  line L18 (-41.6667, 0) -> (-50, 0)
  line L19 (-50, 0) -> (-50, -3)
  line L20 (-50, -3) -> (-72, -3)
  line L21 (-72, -3) -> (-72, -22.5)
  line L22 (-72, -22.5) -> (-75, -22.5)
  line L23 (-75, -22.5) -> (-75, -32.1429)
  line L24 (-75, -32.1429) -> (-72, -32.1429)
  line L25 (-72, -32.1429) -> (-72, -42.8571)
  line L26 (-72, -42.8571) -> (-75, -42.8571)
  line L27 (-75, -42.8571) -> (-75, -52.5)
  line L28 (-37.5, -72) -> (-37.5, -3) construction
  line L29 (-3, -37.5) -> (-72, -37.5) construction
  line L30 (-31.5, -48.875) -> (-43.5, -48.875)
  line L31 (-43.5, -48.875) -> (-43.5, -26.125)
  line L32 (-43.5, -26.125) -> (-31.5, -26.125)
  line L33 (-31.5, -26.125) -> (-31.5, -48.875)
  line L34 (-31.5, -48.875) -> (-43.5, -26.125) construction
  line L35 (-43.5, -48.875) -> (-31.5, -26.125) construction
  line L36 (-12.5, -63.875) -> (-62.5, -63.875)
  line L37 (-62.5, -63.875) -> (-62.5, -53.875)
  line L38 (-12.5, -53.875) -> (-12.5, -63.875)
  line L39 (-12.5, -53.875) -> (-62.5, -53.875)
  line L40 (-31.5, -48.875) -> (-43.5, -48.875)
  line L41 (-43.5, -48.875) -> (-43.5, -53.875)
  line L42 (-43.5, -53.875) -> (-31.5, -53.875)
  line L43 (-31.5, -53.875) -> (-31.5, -48.875)
  point P0 (-37.5, -37.5)
  dimension "d148" = 22.75
  dimension "d150" = 50
  dimension "d153" = 10
  dimension "d154" = 5
  constraint midpoint L2 L28.start
  constraint midpoint L16 L28.end
  constraint midpoint L7 L29.start
  constraint midpoint L25 L29.end
  constraint horizontal L30
  constraint perpendicular L30 L31
  constraint parallel L30 L32
  constraint parallel L31 L33
  constraint coincident L34 P0
  constraint coincident L35 P0
  constraint midpoint L29 P0
  constraint horizontal L36
  constraint vertical L37
  constraint vertical L38
  constraint perpendicular L37 L39
  constraint horizontal L40
  constraint vertical L41
  constraint horizontal L42
  constraint vertical L43
  constraint coincident L30.end L31.start
  constraint midpoint L39 L42
  measures "d148" distance of L30.end L31.end
  measures "d150" distance of L36.start L36.end
  measures "d153" distance of L36.start L38.start
  measures "d154" distance of L30.end L41.end
extrude "Extrude5''" cut sketch "Sketch3" against normal blind 17 contours L30 L39 L40 L41 L42 L43 | L30 L31 L32 L33 L40 | L36 L37 L38 L39 L42 bodies 6 in component "mid panel"
sketch "Sketch2" plane through (0, 0, 0) normal (0, -1, 0) x (1, 0, 0) in component "front"
  line L0 (25, 127) -> (25, 130)
  line L1 (25, 130) -> (22.5, 130)
  line L2 (22.5, 130) -> (22.5, 200)
  line L3 (22.5, 200) -> (0, 200)
  line L4 (0, 200) -> (0, 177.7778)
  line L5 (0, 177.7778) -> (3, 177.7778)
  line L6 (3, 177.7778) -> (3, 155.5556)
  line L7 (3, 155.5556) -> (0, 155.5556)
  line L8 (0, 155.5556) -> (0, 133.3333)
  line L9 (0, 133.3333) -> (3, 133.3333)
  line L10 (3, 133.3333) -> (3, 111.1111)
  line L11 (3, 111.1111) -> (0, 111.1111)
  line L12 (0, 111.1111) -> (0, 88.8889)
  line L13 (0, 88.8889) -> (3, 88.8889)
  line L14 (3, 88.8889) -> (3, 66.6667)
  line L15 (3, 66.6667) -> (0, 66.6667)
  line L16 (0, 66.6667) -> (0, 44.4444)
  line L17 (0, 44.4444) -> (3, 44.4444)
  line L18 (3, 44.4444) -> (3, 22.2222)
  line L19 (3, 22.2222) -> (0, 22.2222)
  line L20 (0, 22.2222) -> (0, 3)
  line L21 (0, 3) -> (8.3333, 3)
  line L22 (8.3333, 3) -> (8.3333, 0)
  line L23 (8.3333, 0) -> (16.6667, 0)
  line L24 (16.6667, 0) -> (16.6667, 3)
  line L25 (16.6667, 3) -> (25, 3)
  line L26 (25, 3) -> (25, 0)
  line L27 (25, 0) -> (33.3333, 0)
  line L28 (33.3333, 0) -> (33.3333, 3)
  line L29 (33.3333, 3) -> (41.6667, 3)
  line L30 (41.6667, 3) -> (41.6667, 0)
  line L31 (41.6667, 0) -> (50, 0)
  line L32 (50, 0) -> (50, 3)
  line L33 (50, 3) -> (58.3333, 3)
  line L34 (58.3333, 3) -> (58.3333, 0)
  line L35 (58.3333, 0) -> (66.6667, 0)
  line L36 (66.6667, 0) -> (66.6667, 3)
  line L37 (66.6667, 3) -> (75, 3)
  line L38 (75, 3) -> (75, 22.2222)
  line L39 (75, 22.2222) -> (72, 22.2222)
  line L40 (72, 22.2222) -> (72, 44.4444)
  line L41 (72, 44.4444) -> (75, 44.4444)
  line L42 (75, 44.4444) -> (75, 66.6667)
  line L43 (75, 66.6667) -> (72, 66.6667)
  line L44 (72, 66.6667) -> (72, 88.8889)
  line L45 (72, 88.8889) -> (75, 88.8889)
  line L46 (75, 88.8889) -> (75, 111.1111)
  line L47 (75, 111.1111) -> (72, 111.1111)
  line L48 (72, 111.1111) -> (72, 133.3333)
  line L49 (72, 133.3333) -> (75, 133.3333)
  line L50 (75, 133.3333) -> (75, 155.5556)
  line L51 (75, 155.5556) -> (72, 155.5556)
  line L52 (72, 155.5556) -> (72, 177.7778)
  line L53 (72, 177.7778) -> (75, 177.7778)
  line L54 (75, 177.7778) -> (75, 200)
  line L55 (75, 200) -> (52.5, 200)
  line L56 (52.5, 200) -> (52.5, 130)
  line L57 (52.5, 130) -> (50, 130)
  line L58 (50, 130) -> (50, 127)
  line L59 (50, 127) -> (41.6667, 127)
  line L60 (41.6667, 127) -> (41.6667, 130)
  line L61 (41.6667, 130) -> (33.3333, 130)
  line L62 (33.3333, 130) -> (33.3333, 127)
  line L63 (33.3333, 127) -> (25, 127)
  line L64 (22.5, 200) -> (52.5, 200)
  line L65 (52.5, 200) -> (52.5, 156)
  line L66 (52.5, 156) -> (22.5, 156)
  line L67 (22.5, 156) -> (22.5, 200)
  dimension "d155" = 26
  constraint horizontal L64
  constraint vertical L65
  constraint horizontal L66
  constraint vertical L67
  constraint coincident L56 L65.end
  constraint coincident L2.end L3.start
  measures "d155" distance of L61 L66
extrude "Extrude4''" add sketch "Sketch2" against normal blind 3 contours L2 L56 L64 L65 L66 L67 bodies 3 in component "front"
sketch "Sketch6" plane through (72, 0, 0) normal (-1, 0, 0) x (0, -1, 0) in component "right"
  line L0 (-75, 66.6667) -> (-72, 66.6667)
  line L1 (-72, 3) -> (-64.2857, 3)
  line L2 (-64.2857, 3) -> (-64.2857, 0)
  line L3 (-64.2857, 0) -> (-53.5714, 0)
  line L4 (-53.5714, 0) -> (-53.5714, 3)
  line L5 (-53.5714, 3) -> (-42.8571, 3)
  line L6 (-42.8571, 3) -> (-42.8571, 0)
  line L7 (-42.8571, 0) -> (-32.1429, 0)
  line L8 (-32.1429, 0) -> (-32.1429, 3)
  line L9 (-32.1429, 3) -> (-21.4286, 3)
  line L10 (-21.4286, 3) -> (-21.4286, 0)
  line L11 (-21.4286, 0) -> (-10.7143, 0)
  line L12 (-10.7143, 0) -> (-10.7143, 3)
  line L13 (-10.7143, 3) -> (-3, 3)
  line L14 (-3, 3) -> (-3, 22.2222)
  line L15 (-3, 22.2222) -> (0, 22.2222)
  line L16 (0, 22.2222) -> (0, 44.4444)
  line L17 (0, 44.4444) -> (-3, 44.4444)
  line L18 (-3, 44.4444) -> (-3, 66.6667)
  line L19 (-3, 66.6667) -> (0, 66.6667)
  line L20 (0, 66.6667) -> (0, 88.8889)
  line L21 (0, 88.8889) -> (-3, 88.8889)
  line L22 (-3, 88.8889) -> (-3, 111.1111)
  line L23 (-3, 111.1111) -> (0, 111.1111)
  line L24 (0, 111.1111) -> (0, 133.3333)
  line L25 (0, 133.3333) -> (-3, 133.3333)
  line L26 (-3, 133.3333) -> (-3, 155.5556)
  line L27 (-3, 155.5556) -> (0, 155.5556)
  line L28 (0, 155.5556) -> (0, 177.7778)
  line L29 (0, 177.7778) -> (-3, 177.7778)
  line L30 (-3, 177.7778) -> (-3, 200)
  line L31 (-3, 200) -> (-22.5, 200)
  line L32 (-22.5, 200) -> (-22.5, 127)
  line L33 (-22.5, 127) -> (-32.1429, 127)
  line L34 (-32.1429, 127) -> (-32.1429, 130)
  line L35 (-32.1429, 130) -> (-42.8571, 130)
  line L36 (-42.8571, 130) -> (-42.8571, 127)
  line L37 (-42.8571, 127) -> (-52.5, 127)
  line L38 (-52.5, 127) -> (-52.5, 200)
  line L39 (-52.5, 200) -> (-72, 200)
  line L40 (-72, 66.6667) -> (-72, 3)
  line L41 (-72, 177.7778) -> (-75, 177.7778)
  line L42 (-75, 177.7778) -> (-75, 155.5556)
  line L43 (-75, 155.5556) -> (-72, 155.5556)
  line L44 (-72, 155.5556) -> (-72, 133.3333)
  line L45 (-72, 133.3333) -> (-75, 133.3333)
  line L46 (-75, 133.3333) -> (-75, 111.1111)
  line L47 (-75, 111.1111) -> (-72, 111.1111)
  line L48 (-72, 111.1111) -> (-72, 88.8889)
  line L49 (-72, 88.8889) -> (-75, 88.8889)
  line L50 (-75, 88.8889) -> (-75, 66.6667)
  line L51 (-52.5, 200) -> (-22.5, 200)
  line L52 (-22.5, 200) -> (-22.5, 104)
  line L53 (-22.5, 104) -> (-52.5, 104)
  line L54 (-52.5, 104) -> (-52.5, 200)
  line L55 (-72, 200) -> (-72, 177.7778)
  dimension "d158" = 26
  constraint horizontal L51
  constraint vertical L52
  constraint horizontal L53
  constraint vertical L54
  constraint coincident L32 L52.end
  constraint coincident L38.end L39.start
  measures "d158" distance of L35 L53
extrude "Extrude7" add sketch "Sketch6" against normal blind 3 contours L32 L33 L34 L35 L36 L37 L38 L51 L52 L54 | L33 L34 L35 L36 L37 L52 L53 L54 bodies 4 in component "right"